Autodesk Fusion 360 part; units mm, degrees
(part 2 of 2)
sketch "Sketch1" plane through (0, 0, 0) normal (0, 1, 0) x (1, 0, 0)
  line L0 (-3.0515, -3.9) -> (3.0515, -3.9)
  line L1 (3.9, -3.0515) -> (3.9, 3.0515)
  line L2 (3.0515, 3.9) -> (-3.0515, 3.9)
  line L3 (-3.9, 3.0515) -> (-3.9, -3.0515)
  line L4 (10, -10) -> (3.9, -3.9) construction
  line L5 (-3.9, 3.9) -> (-10, 10) construction
  line L6 (3.9, 3.9) -> (10, 10) construction
  line L7 (-3.1, -9.5) -> (-3.1, -8.2)
  line L8 (-3.6, -10) -> (-10, -10)
  line L9 (-10, -10) -> (-10, -8.2)
  line L10 (-3.1, -8.2) -> (-3.1, -9.5)
  line L11 (-10, -10) -> (-8.2, -10)
  line L12 (-8.2, -3.1) -> (-9.5, -3.1)
  line L13 (-10, -3.6) -> (-10, -10)
  line L14 (-10, -10) -> (-5.5, -10)
  line L15 (-5.5, -8.2) -> (-5.5, -6.3485)
  line L16 (-6.3485, -5.5) -> (-8.2, -5.5)
  line L17 (-8.2, -5.5) -> (-8.2, -3.1)
  line L18 (-5.5, -8.2) -> (-3.1, -8.2)
  line L19 (0, 0) -> (10.4977, 0) construction
  line L20 (-3.9, -3.0515) -> (-6.3485, -5.5)
  line L21 (-3.0515, -3.9) -> (-5.5, -6.3485)
  line L22 (-3.6, -10) -> (-3.6, -9.5)
  line L23 (-3.6, -9.5) -> (-3.1, -9.5)
  line L24 (-10, -10) -> (-3.6, -10)
  line L25 (-9.5, -3.1) -> (-9.5, -3.6)
  line L26 (-9.5, -3.6) -> (-10, -3.6)
  line L27 (-10, -3.6) -> (-10, -10)
  line L28 (-10, 10) -> (-3.6, 10)
  line L29 (-9.5, 3.1) -> (-9.5, 3.6)
  line L30 (-10, 10) -> (-5.5, 10)
  line L31 (-3.0515, 3.9) -> (-5.5, 6.3485)
  line L32 (-10, 3.6) -> (-10, 10)
  line L33 (-3.6, 10) -> (-3.6, 9.5)
  line L34 (-9.5, 3.6) -> (-10, 3.6)
  line L35 (-3.6, 9.5) -> (-3.1, 9.5)
  line L36 (-3.9, 3.0515) -> (-6.3485, 5.5)
  line L37 (-8.2, 5.5) -> (-8.2, 3.1)
  line L38 (-5.5, 8.2) -> (-3.1, 8.2)
  line L39 (-10, 10) -> (-8.2, 10)
  line L40 (-10, 10) -> (-10, 8.2)
  line L41 (-10, 3.6) -> (-10, 10)
  line L42 (-5.5, 8.2) -> (-5.5, 6.3485)
  line L43 (-6.3485, 5.5) -> (-8.2, 5.5)
  line L44 (-3.6, 10) -> (-10, 10)
  line L45 (-8.2, 3.1) -> (-9.5, 3.1)
  line L46 (-3.1, 8.2) -> (-3.1, 9.5)
  line L47 (10, 10) -> (8.2, 10)
  line L48 (5.5, 8.2) -> (3.1, 8.2)
  line L49 (10, 10) -> (10, 8.2)
  line L50 (3.1, 8.2) -> (3.1, 9.5)
  line L51 (5.5, 8.2) -> (5.5, 6.3485)
  line L52 (10, 3.6) -> (10, 10)
  line L53 (6.3485, 5.5) -> (8.2, 5.5)
  line L54 (8.2, 5.5) -> (8.2, 3.1)
  line L55 (10, 10) -> (5.5, 10)
  line L56 (9.5, 3.1) -> (9.5, 3.6)
  line L57 (8.2, 3.1) -> (9.5, 3.1)
  line L58 (3.6, 10) -> (10, 10)
  line L59 (3.0515, 3.9) -> (5.5, 6.3485)
  line L60 (10, 3.6) -> (10, 10)
  line L61 (9.5, 3.6) -> (10, 3.6)
  line L62 (3.6, 10) -> (3.6, 9.5)
  line L63 (3.9, 3.0515) -> (6.3485, 5.5)
  line L64 (3.6, 9.5) -> (3.1, 9.5)
  line L65 (10, 10) -> (3.6, 10)
  line L66 (3.9, 3.9) -> (10, 10) construction
  line L67 (3.6, -9.5) -> (3.1, -9.5)
  line L68 (10, -3.6) -> (10, -10)
  line L69 (9.5, -3.6) -> (10, -3.6)
  line L70 (9.5, -3.1) -> (9.5, -3.6)
  line L71 (10, -10) -> (3.6, -10)
  line L72 (5.5, -8.2) -> (5.5, -6.3485)
  line L73 (8.2, -3.1) -> (9.5, -3.1)
  line L74 (10, -10) -> (8.2, -10)
  line L75 (10, -3.6) -> (10, -10)
  line L76 (3.0515, -3.9) -> (5.5, -6.3485)
  line L77 (3.1, -8.2) -> (3.1, -9.5)
  line L78 (6.3485, -5.5) -> (8.2, -5.5)
  line L79 (10, -10) -> (10, -8.2)
  line L80 (3.9, -3.0515) -> (6.3485, -5.5)
  line L81 (3.6, -10) -> (3.6, -9.5)
  line L82 (8.2, -5.5) -> (8.2, -3.1)
  line L83 (5.5, -8.2) -> (3.1, -8.2)
  line L84 (10, -10) -> (5.5, -10)
  line L85 (3.1, -9.5) -> (3.1, -8.2)
  line L86 (3.6, -10) -> (10, -10)
extrude "Extrude1" add sketch "Sketch1" along normal blind 150
sketch "Sketch2" plane through (0, 150, 0) normal (0, 1, 0) x (-1, 0, 0)
  line L0 (-3.6, 9.5) -> (-3.6, 10)
  line L1 (-3.6, 10) -> (-10, 10)
  line L2 (-10, 10) -> (-10, 3.6)
  line L3 (-10, 3.6) -> (-9.5, 3.6)
  line L4 (-9.5, 3.6) -> (-9.5, 3.1)
  line L5 (-9.5, 3.1) -> (-8.2, 3.1)
  line L6 (-8.2, 3.1) -> (-8.2, 5.5)
  line L7 (-8.2, 5.5) -> (-6.3485, 5.5)
  line L8 (-6.3485, 5.5) -> (-3.9, 3.0515)
  line L9 (-3.9, 3.0515) -> (-3.9, -3.0515)
  line L10 (-3.9, -3.0515) -> (-6.3485, -5.5)
  line L11 (-6.3485, -5.5) -> (-8.2, -5.5)
  line L12 (-8.2, -5.5) -> (-8.2, -3.1)
  line L13 (-8.2, -3.1) -> (-9.5, -3.1)
  line L14 (-9.5, -3.1) -> (-9.5, -3.6)
  line L15 (-9.5, -3.6) -> (-10, -3.6)
  line L16 (-10, -3.6) -> (-10, -10)
  line L17 (-10, -10) -> (-3.6, -10)
  line L18 (-3.6, -10) -> (-3.6, -9.5)
  line L19 (-3.6, -9.5) -> (-3.1, -9.5)
  line L20 (-3.1, -9.5) -> (-3.1, -8.2)
  line L21 (-3.1, -8.2) -> (-5.5, -8.2)
  line L22 (-5.5, -8.2) -> (-5.5, -6.3485)
  line L23 (-5.5, -6.3485) -> (-3.0515, -3.9)
  line L24 (-3.0515, -3.9) -> (3.0515, -3.9)
  line L25 (3.0515, -3.9) -> (5.5, -6.3485)
  line L26 (5.5, -6.3485) -> (5.5, -8.2)
  line L27 (5.5, -8.2) -> (3.1, -8.2)
  line L28 (3.1, -8.2) -> (3.1, -9.5)
  line L29 (3.1, -9.5) -> (3.6, -9.5)
  line L30 (3.6, -9.5) -> (3.6, -10)
  line L31 (3.6, -10) -> (10, -10)
  line L32 (10, -10) -> (10, -3.6)
  line L33 (10, -3.6) -> (9.5, -3.6)
  line L34 (9.5, -3.6) -> (9.5, -3.1)
  line L35 (9.5, -3.1) -> (8.2, -3.1)
  line L36 (8.2, -3.1) -> (8.2, -5.5)
  line L37 (8.2, -5.5) -> (6.3485, -5.5)
  line L38 (6.3485, -5.5) -> (3.9, -3.0515)
  line L39 (3.9, -3.0515) -> (3.9, 3.0515)
  line L40 (3.9, 3.0515) -> (6.3485, 5.5)
  line L41 (6.3485, 5.5) -> (8.2, 5.5)
  line L42 (8.2, 5.5) -> (8.2, 3.1)
  line L43 (8.2, 3.1) -> (9.5, 3.1)
  line L44 (9.5, 3.1) -> (9.5, 3.6)
  line L45 (9.5, 3.6) -> (10, 3.6)
  line L46 (10, 3.6) -> (10, 10)
  line L47 (10, 10) -> (3.6, 10)
  line L48 (3.6, 10) -> (3.6, 9.5)
  line L49 (3.6, 9.5) -> (3.1, 9.5)
  line L50 (3.1, 9.5) -> (3.1, 8.2)
  line L51 (3.1, 8.2) -> (5.5, 8.2)
  line L52 (5.5, 8.2) -> (5.5, 6.3485)
  line L53 (5.5, 6.3485) -> (3.0515, 3.9)
  line L54 (3.0515, 3.9) -> (-3.0515, 3.9)
  line L55 (-3.0515, 3.9) -> (-5.5, 6.3485)
  line L56 (-5.5, 6.3485) -> (-5.5, 8.2)
  line L57 (-5.5, 8.2) -> (-3.1, 8.2)
  line L58 (-3.1, 8.2) -> (-3.1, 9.5)
  line L59 (-3.1, 9.5) -> (-3.6, 9.5)
  circle A0 centre (0, 0) radius 2.5
  dimension "d25" = 5
  measures "d25" diameter of A0
extrude "Extrude2" cut sketch "Sketch2" against normal through all contours A0
fillet "Fillet1" radius 0.5 4 edges at (-10, 75, -10) (-10, 75, 10) (10, 75, 10) (10, 75, -10)

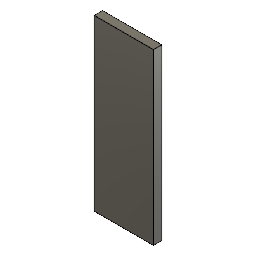
design "chapa-metalica"
Autodesk Fusion 360 part; units mm, degrees
sketch "Sketch1" plane through (0, 0, 0) normal (0, 1, 0) x (1, 0, 0)
  line L0 (-31.9947, -5) -> (28.0053, -5)
  line L1 (28.0053, -5) -> (28.0053, 5)
  line L2 (28.0053, 5) -> (-31.9947, 5)
  line L3 (-31.9947, 5) -> (-31.9947, -5)
  line L4 (-31.9947, -5) -> (28.0053, 5) construction
  line L5 (28.0053, -5) -> (-31.9947, 5) construction
  dimension "d1" = 60
  dimension "d2" = 10
extrude "Extrude1" add sketch "Sketch1" along normal blind 200
move_face "OffsetFaces1" offset 10 1 faces at (28.0053, 66.6667, 1.6667)
